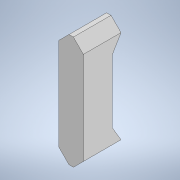
# Autodesk Inventor part: LegConnectorBase
Saved by Autodesk Inventor 2022 (Build 260153000, 153)
## iProperties
Created: 2021-12-19
Part Number: LegConnectorBase
Material: Generic
Document SubType Name: Modeling
Designer: dangl
Density: 1 g/cm^3
Appearance: Default
Author: dangl
Autodesk Inventor part; units mm, degrees
ref_plane "YZ Plane" through (0, 0, 0) normal (1, 0, 0) x (0, 1, 0)
ref_plane "XZ Plane" through (0, 0, 0) normal (0, 1, 0) x (-1, 0, 0)
sketch "Sketch1" plane through (0, 0, 0) normal (1, 0, 0) x (0, 1, 0)
  line L0 (2.625, 15.2971) -> (2.625, 13.1655) projected
  line L1 (2.625, 13.1655) -> (3.1907, 13.1655) projected
  line L2 (3.1907, 13.1655) -> (3.1907, 15.2971) projected
  line L3 (3.1907, 15.2971) -> (2.625, 15.2971) projected
  point P0 (0, 0)
ref_plane "Work Plane2" through (0, 2.625, 13.1655) normal (0, 0, 1) x (1, 0, 0)
ref_plane "Work Plane1" through (0, 0, 0) normal (0, 0, 1) x (1, 0, 0)
sketch "Sketch2" plane through (0, 2.625, 13.1655) normal (0, 0, 1) x (1, 0, 0)
  line L0 (-0.6907, 0) -> (-0.125, 0.5657) projected
  line L1 (0.6907, 0) -> (0.125, 0.5657) projected
  line L2 (-0.6907, -5.25) -> (-0.125, -5.8157) projected
  line L3 (0.6907, -5.25) -> (0.125, -5.8157) projected
  line L4 (-0.6907, 0) -> (-0.6907, -5.25)
  line L5 (-0.125, -5.8157) -> (0.125, -5.8157)
  line L6 (0.6907, -5.25) -> (0.6907, 0)
  line L7 (0.125, 0.5657) -> (-0.125, 0.5657)
  point P0 (0, -2.625)
  constraints: 8 end point, 3 perpendicular, 1 point on line, 1 vertical
extrude "Extrusion1" add sketch "Sketch2" along normal up to surface (2.1316 mm away)
sketch "Sketch3" plane through (0.6907, -2.625, 13.1655) normal (1, 0, 0) x (0, 0, -1)
  line L0 (0, 5.25) -> (-2.3345, 8.1092) projected
  line L1 (0, 5.25) -> (0, 5.8157) projected
  line L2 (0, 5.25) -> (-0.5, 4.4102)
  line L3 (0, 5.25) -> (0, 0) projected
  line L4 (0, 2.625) -> (-0.5, 2.625)
  line L5 (0, 0) -> (-0.5, 0.8398)
  line L6 (0, 5.25) -> (-2.1316, 5.25) projected
  line L7 (0, 5.25) -> (0, 0)
  line L8 (-0.5, 0.8398) -> (-0.5, 4.4102)
  point P0 (13.1655, 2.625)
  dimension "d2" = 110
  dimension "d3" = 0.5
  constraints: 10 end point, 2 perpendicular, 1 midpoint, 1 parallel, 1 symmetric about line
  measures "d2" angle of L0 L2
  measures "d3" horizontal distance of L0.start L2.end
extrude "Extrusion2" cut sketch "Sketch3" against normal blind 10
body "Solid1"
